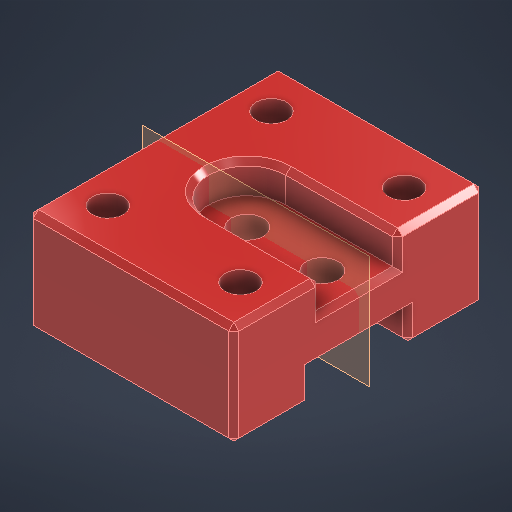
# Autodesk Inventor part: load_cell_connector_top
Saved by Autodesk Inventor 2026 (Build 300175000, 175)
## iProperties
Created: 2025-04-21
Part Number: load_cell_connector_top
Material: Generic
Document SubType Name: Modeling
Designer: Paul Juschitz
Density: 1 g/cm^3
Appearance: Orange-Red
Author: Paul Juschitz
Autodesk Inventor part; units mm, degrees
ref_plane "YZ Plane" through (0, 0, 0) normal (1, 0, 0) x (0, 1, 0)
ref_plane "XZ Plane" through (0, 0, 0) normal (0, 1, 0) x (-1, 0, 0)
ref_plane "XY Plane" through (0, 0, 0) normal (0, 0, 1) x (1, 0, 0)
sketch "Sketch1" plane through (0, 0, 0) normal (0, 1, 0) x (-1, 0, 0)
  circle A0 centre (7.3, 0) radius 1.55
  circle A1 centre (0, 0) radius 1.55
  line L0 (0, 10.8163) -> (0, -10.8163)
  line L1 (6.335, 0) -> (-6.335, 0)
  line L2 (-3.55, 12.16) -> (16.45, 12.16)
  line L3 (16.45, 12.16) -> (16.45, -12.16)
  line L4 (16.45, -12.16) -> (-3.55, -12.16)
  line L5 (-3.55, -12.16) -> (-3.55, 12.16)
  dimension "d0" = 3.1
  dimension "d1" = 7.3
  dimension "d2" = 2
  dimension "d3" = 24.32
  dimension "d4" = 20
  constraints: 12 end point, 2 centre point, 2 horizontal, 2 midpoint, 2 parallel, 2 symmetric about line, 1 equal radius, 1 perpendicular, 1 point on line, 1 vertical
  measures "d0" diameter of A0
  measures "d1" distance of A1.centre A0.centre
  measures "d2" distance edge to line of A1 L5
  measures "d3" distance of L4.end L2.start
  measures "d4" distance of L2.start L2.end
extrude "Extrusion1" add sketch "Sketch1" along normal blind 10
sketch "Sketch2" plane through (0, 0, 0) normal (0, -1, 0) x (1, 0, 0)
  line L0 (3.55, 4.76) -> (-11.68, 4.76)
  line L1 (-11.68, 4.76) -> (-11.68, -4.76)
  line L2 (-11.68, -4.76) -> (3.55, -4.76)
  line L3 (3.55, -4.76) -> (3.55, 4.76)
  circle A0 centre (0, 0) radius 1.55 projected
  circle A1 centre (-7.3, 0) radius 1.55 projected
  line L4 (0, 0) -> (-7.3, 0)
  line L5 (3.55, 12.16) -> (3.55, -12.16) projected
  dimension "d7" = 9.52
  dimension "d8" = 4.38
  constraints: 10 end point, 2 horizontal, 2 parallel, 1 coincident, 1 perpendicular, 1 point on line, 1 other
  measures "d7" distance of L0.end L1.end
  measures "d8" distance from line of L1 L4.end
extrude "Extrusion2" cut sketch "Sketch2" against normal blind 3
sketch "Sketch3" plane through (0, 10, 0) normal (0, 1, 0) x (1, 0, 0)
  circle A0 centre (-7.3, 0) radius 1.55 projected
  circle A1 centre (0, 0) radius 1.55 projected
  arc A2 (3.55, -1.2083) -> (3.55, 1.2083) centre (0, 0) ccw
  arc A3 (-7.3, 3.75) -> (-7.3, -3.75) centre (-7.3, 0) ccw
  line L0 (3.55, -12.16) -> (3.55, 12.16) projected
  line L1 (-7.3, 3.75) -> (0, 3.75)
  line L2 (-7.3, -3.75) -> (0, -3.75)
  line L3 (3.55, -1.2083) -> (3.55, 1.2083)
  line L4 (3.55, -1.2083) -> (3.55, 1.2083)
  line L5 (0, -3.75) -> (3.55, -3.75)
  line L6 (0, 3.75) -> (3.55, 3.75)
  dimension "d11" = 7.5
  constraints: 12 end point, 5 tangent, 4 point on circle, 4 point on line, 2 centre point, 2 coincident, 2 perpendicular, 1 collinear, 1 equal radius
  measures "d11" diameter of A2
extrude "Extrusion3" cut sketch "Sketch3" against normal blind 3 contours L0 L5 L2 A3 L1 L6
sketch "Sketch4" plane through (0, 10, 0) normal (0, 1, 0) x (1, 0, 0)
  line L0 (3.55, -12.16) -> (3.55, -3.75) projected
  line L1 (3.55, -3.75) -> (-7.3, -3.75) projected
  arc A0 (-7.3, 3.75) -> (-7.3, -3.75) centre (-7.3, 0) ccw projected
  line L2 (-7.3, 3.75) -> (3.55, 3.75) projected
  line L3 (3.55, 3.75) -> (3.55, -3.75) projected
  circle A1 centre (0, -7.955) radius 1.5
  circle A2 centre (-12.9, -7.955) radius 1.5
  line L4 (-16.45, 12.16) -> (-16.45, -12.16) projected
  line L5 (-16.45, 0) -> (3.55, 0)
  circle A3 centre (0, 7.955) radius 1.5
  circle A4 centre (-12.9, 7.955) radius 1.5
  line L6 (3.55, -7.955) -> (-16.45, -7.955)
  line L7 (3.55, 4.76) -> (3.55, 12.16) projected
  line L8 (3.55, 7.955) -> (-16.45, 7.955)
  line L9 (-11.05, 0) -> (-16.45, 0) construction
  point P0 (0, 0)
  dimension "d15" = 3
  dimension "d16" = 3
  dimension "d18" = 3.55
  dimension "d19" = 3.55
  constraints: 8 end point, 5 point on line, 4 centre point, 3 midpoint, 3 perpendicular, 2 symmetric about line, 1 horizontal alignment, 1 point on circle, 1 vertical alignment, 3 other
  measures "d15" diameter of A1
  measures "d16" diameter of A2
  measures "d18" distance from line of L0 A1.centre
  measures "d19" distance from line of L4 A2.centre
extrude "Extrusion4" cut sketch "Sketch4" against normal blind 5 contours L6 A1 | A1 L6 | L6 A2 | A2 L6 | L8 A3 | A3 L8 | L8 A4 | A4 L8
chamfer "Chamfer1" distance 0.5 angle 45 26 edges at (3.55, 10, 7.955) (-1.875, 10, 3.75) (-11.05, 10, 0) (-1.875, 10, -3.75) (3.55, 10, -7.955) (-6.45, 10, -12.16) (-16.45, 10, 0) (-6.45, 10, 12.16) (3.55, 5, 12.16) (3.55, 0, 8.46) (-6.45, 0, 12.16) (-16.45, 0, 0) (-6.45, 0, -12.16) (3.55, 0, -8.46) (3.55, 5, -12.16) (-16.45, 5, -12.16) (-16.45, 5, 12.16) (-11.68, 0, 0) (-4.065, 0, 4.76) (-4.065, 0, -4.76) (3.55, 1.5, 4.76) (3.55, 1.5, -4.76) (3.55, 3, 0) (3.55, 7, 0) (3.55, 8.5, 3.75) (3.55, 8.5, -3.75)
ref_plane "Work Plane1" through (-15.95, 0.5, 0) normal (0, 0, 1) x (1, 0, 0)
equation "\"d0\" = spacer_hole_diameter"
equation "\"d1\" = load_cell_hole_discance"
equation "\"load_cell_hole_discance\" = 7.3"
equation "\"spacer_hole_diameter\" = 3.1"
equation "\"load_cell_width\" = 9.32"
equation "\"load_cell_hole_edge\" = 4.18"
body "Solid1"
